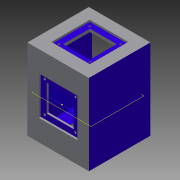
# Autodesk Inventor part: brain box bottom
Saved by Autodesk Inventor 2015 (Build 190159000, 159)
## iProperties
Created: 2014-09-09
Part Number: brain box bottom
Material: Generic
Document SubType Name: Modeling
Designer: ericd_000
Density: 1 g/cm^3
Appearance: Default
Author: ericd_000
Autodesk Inventor part; units mm, degrees
ref_plane "YZ Plane" through (0, 0, 0) normal (1, 0, 0) x (0, 1, 0)
ref_plane "XZ Plane" through (0, 0, 0) normal (0, 1, 0) x (-1, 0, 0)
ref_plane "XY Plane" through (0, 0, 0) normal (0, 0, 1) x (1, 0, 0)
sketch "Sketch1" plane through (0, 0, 0) normal (0, 1, 0) x (-1, 0, 0)
  line L0 (80, 100) -> (-80, 100)
  line L1 (-80, 100) -> (-80, -100)
  line L2 (-80, -100) -> (80, -100)
  line L3 (80, -100) -> (80, 100)
  point P0 (0, 0)
  point P1 (80, 0)
  point P2 (0, -100)
  dimension "d0" = 200
  dimension "d1" = 160
  constraints: 8 end point, 2 midpoint, 2 parallel, 1 horizontal, 1 horizontal alignment, 1 perpendicular, 1 vertical alignment
  measures "d0" distance of L2.end L0.start
  measures "d1" distance of L0.start L0.end
extrude "Extrusion1" add sketch "Sketch1" along normal blind 5
sketch "Sketch2" plane through (0, 5, 0) normal (0, 1, 0) x (1, 0, 0)
  line L0 (-80, -100) -> (80, -100)
  line L1 (80, -100) -> (80, 100)
  line L2 (80, 100) -> (-80, 100)
  line L3 (-80, 100) -> (-80, -100)
  line L4 (-72, -92) -> (72, -92)
  line L5 (72, -92) -> (72, 92)
  line L6 (72, 92) -> (-72, 92)
  line L7 (-72, 92) -> (-72, -92)
  point P0 (0, 0)
  dimension "d4" = 8
  constraints: 16 end point, 4 parallel, 2 perpendicular, 1 horizontal, 3 other
  measures "d4" distance between parallel lines of L3 L7
extrude "Extrusion2" add sketch "Sketch2" along normal blind 150
sketch "Sketch3" plane through (0, 155, 0) normal (0, 1, 0) x (1, 0, 0)
  circle A0 centre (-76, 96) radius 1.5
  circle A1 centre (76, 96) radius 1.5
  circle A2 centre (76, -96) radius 1.5
  circle A3 centre (-76, -96) radius 1.5
  line L0 (80, -100) -> (80, 100) projected
  line L1 (-80, -100) -> (80, -100) projected
  line L2 (80, 100) -> (-80, 100) projected
  line L3 (-80, 100) -> (-80, -100) projected
  point P0 (0, 0)
  dimension "d8" = 3
  dimension "d12" = 4
  dimension "d16" = 4
  dimension "d18" = 3
  dimension "d19" = 4
  dimension "d20" = 4
  dimension "d21" = 3
  dimension "d22" = 4
  dimension "d23" = 4
  dimension "d24" = 4
  dimension "d25" = 4
  dimension "d26" = 3
  constraints: 4 centre point
  measures "d8" diameter of A1
  measures "d12" distance from line of A1.centre L0
  measures "d16" distance from line of L2 A1.centre
  measures "d18" diameter of A0
  measures "d19" distance from line of L3 A0.centre
  measures "d20" distance from line of L2 A0.centre
  measures "d21" diameter of A2
  measures "d22" distance from line of L0 A2.centre
  measures "d23" distance from line of L1 A2.centre
  measures "d24" distance from line of L3 A3.centre
  measures "d25" distance from line of A3.centre L1
  measures "d26" diameter of A3
extrude "Extrusion3" cut sketch "Sketch3" against normal blind 15 contours A0 | A1 | A2 | A3
sketch "Sketch4" plane through (80, 0, 100) normal (1, 0, 0) x (0, 0, -1)
  line L0 (50, 127.5) -> (150, 127.5)
  line L1 (150, 127.5) -> (150, 27.5)
  line L2 (150, 27.5) -> (50, 27.5)
  line L3 (50, 27.5) -> (50, 127.5)
  line L4 (0, 155) -> (200, 155) projected
  line L5 (200, 0) -> (200, 155) projected
  point P0 (100, 0)
  point P1 (100, 127.5)
  point P2 (100, 155)
  point P3 (150, 77.5)
  point P4 (200, 77.5)
  dimension "d29" = 100
  dimension "d30" = 100
  constraints: 8 end point, 4 midpoint, 2 parallel, 1 horizontal, 1 horizontal alignment, 1 perpendicular, 1 vertical alignment
  measures "d29" distance of L0.start L0.end
  measures "d30" distance of L2.end L0.start
sketch "Sketch5" plane through (-80, 0, 100) normal (0, 0, 1) x (1, 0, 0)
  line L0 (45, 112.5) -> (115, 112.5)
  line L1 (115, 112.5) -> (115, 42.5)
  line L2 (115, 42.5) -> (45, 42.5)
  line L3 (45, 42.5) -> (45, 112.5)
  line L4 (160, 0) -> (160, 155) projected
  line L5 (0, 155) -> (160, 155) projected
  point P0 (80, 0)
  point P1 (115, 77.5)
  point P2 (160, 77.5)
  point P3 (80, 112.5)
  point P4 (80, 155)
  dimension "d31" = 70
  dimension "d32" = 70
  constraints: 8 end point, 4 midpoint, 2 parallel, 1 horizontal, 1 horizontal alignment, 1 perpendicular, 1 vertical alignment
  measures "d31" distance of L0.start L0.end
  measures "d32" distance of L0.end L1.end
extrude "Extrusion4" cut sketch "Sketch5" against normal blind 10
sketch "Sketch6" plane through (-80, 0, 100) normal (0, 0, 1) x (1, 0, 0)
  line L0 (45, 112.5) -> (115, 112.5)
  line L1 (115, 112.5) -> (115, 42.5)
  line L2 (115, 42.5) -> (45, 42.5)
  line L3 (45, 42.5) -> (45, 112.5)
  line L4 (30, 127.5) -> (130, 127.5)
  line L5 (130, 127.5) -> (130, 27.5)
  line L6 (130, 27.5) -> (30, 27.5)
  line L7 (30, 27.5) -> (30, 127.5)
  circle A0 centre (40, 117.5) radius 2.75
  circle A1 centre (40, 37.5) radius 2.75
  circle A2 centre (120, 117.5) radius 2.75
  circle A3 centre (120, 37.5) radius 2.75
  point P0 (80, 0)
  dimension "d35" = 15
  dimension "d36" = 10
  dimension "d37" = 10
  dimension "d38" = 5.5
  dimension "d41" = 80
  dimension "d44" = 80
  constraints: 16 end point, 4 centre point, 4 parallel, 2 horizontal, 2 perpendicular, 1 vertical, 9 other
  measures "d35" distance between parallel lines of L4 L0
  measures "d36" distance from line of L7 A0.centre
  measures "d37" distance from line of L4 A0.centre
  measures "d38" diameter of A0
  measures "d41" distance of A0.centre A1.centre
  measures "d44" distance of A0.centre A2.centre
extrude "Extrusion5" cut sketch "Sketch6" against normal blind 8 contours A0 | A1 | A2 | A3
sketch "Sketch7" plane through (0, 5, 0) normal (0, 1, 0) x (1, 0, 0)
  line L0 (72, 92) -> (72, -92) construction
  line L1 (72, 0) -> (-72, 0) construction
  line L2 (-72, -92) -> (-72, 92) construction
  point P0 (0, 0)
  constraints: 2 end point, 2 midpoint
ref_plane "Work Plane1" through (72, 5, 0) normal (0, 0, -1) x (-1, 0, 0)
mirror "Mirror1" about plane through (72, 5, 0) normal (0, 0, -1) of "Extrusion5"
mirror "Mirror2" about plane through (72, 5, 0) normal (0, 0, -1) of "Extrusion4"
sketch "Sketch8" plane through (0, 0, 0) normal (0, -1, 0) x (1, 0, 0)
  line L0 (35, -35) -> (-35, -35)
  line L1 (-35, -35) -> (-35, 35)
  line L2 (-35, 35) -> (35, 35)
  line L3 (35, 35) -> (35, -35)
  line L4 (50, -50) -> (-50, -50)
  line L5 (-50, -50) -> (-50, 50)
  line L6 (-50, 50) -> (50, 50)
  line L7 (50, 50) -> (50, -50)
  circle A0 centre (40, -40) radius 2.75
  circle A1 centre (40, 40) radius 2.75
  circle A2 centre (-40, -40) radius 2.75
  circle A3 centre (-40, 40) radius 2.75
  point P0 (0, 0)
  point P1 (-35, 0)
  point P2 (0, -35)
  dimension "d50" = 70
  dimension "d51" = 70
  dimension "d52" = 15
  dimension "d53" = 5.5
  dimension "d54" = 10
  dimension "d55" = 10
  dimension "d58" = 80
  dimension "d65" = 80
  constraints: 16 end point, 4 centre point, 4 parallel, 2 horizontal, 2 midpoint, 2 perpendicular, 1 horizontal alignment, 1 vertical, 1 vertical alignment, 9 other
  measures "d50" distance of L0.start L0.end
  measures "d51" distance of L0.end L1.end
  measures "d52" distance between parallel lines of L7 L3
  measures "d53" diameter of A0
  measures "d54" distance from line of L7 A0.centre
  measures "d55" distance from line of L4 A0.centre
  measures "d58" distance of A0.centre A1.centre
  measures "d65" distance of A0.centre A2.centre
extrude "Extrusion6" cut sketch "Sketch8" against normal blind 8 contours L0 L1 L2 L3 | A0 | A1 | A2 | A3
sketch "Sketch10" plane through (80, 0, -100) normal (0, 0, -1) x (-1, 0, 0)
  line L0 (130, 127.5) -> (30, 127.5)
  line L1 (30, 127.5) -> (30, 27.5)
  line L2 (30, 27.5) -> (130, 27.5)
  line L3 (130, 27.5) -> (130, 127.5)
  line L4 (0, 155) -> (160, 155) projected
  line L5 (115, 112.5) -> (115, 42.5) projected
  line L6 (115, 42.5) -> (45, 42.5) projected
  line L7 (160, 155) -> (0, 155)
  line L8 (0, 155) -> (0, 0)
  line L9 (0, 0) -> (160, 0)
  line L10 (160, 0) -> (160, 155)
  point P0 (80, 0)
  point P1 (130, 77.5)
  point P2 (115, 77.5)
  point P3 (80, 27.5)
  point P4 (80, 42.5)
  dimension "d72" = 100
  dimension "d73" = 100
  constraints: 16 end point, 4 midpoint, 4 parallel, 2 horizontal, 2 perpendicular, 1 horizontal alignment, 1 vertical alignment
  measures "d72" distance of L2.end L0.start
  measures "d73" distance of L1.end L2.end
extrude "Extrusion7" add sketch "Sketch10" along normal blind 5
mirror "Mirror3" about plane through (72, 5, 0) normal (0, 0, -1) of "Extrusion7"
sketch "Sketch11" plane through (0, 0, 0) normal (0, -1, 0) x (1, 0, 0)
  line L0 (50, 50) -> (-50, 50)
  line L1 (-50, 50) -> (-50, -50)
  line L2 (-50, -50) -> (50, -50)
  line L3 (50, -50) -> (50, 50)
  line L4 (35, 35) -> (35, -35) projected
  line L5 (35, -35) -> (-35, -35) projected
  line L6 (80, 105) -> (-80, 105)
  line L7 (-80, 105) -> (-80, -105)
  line L8 (-80, -105) -> (80, -105)
  line L9 (80, -105) -> (80, 105)
  point P0 (0, 0)
  point P1 (50, 0)
  point P2 (35, 0)
  point P3 (0, -50)
  point P4 (0, -35)
  dimension "d77" = 100
  dimension "d78" = 100
  constraints: 16 end point, 4 midpoint, 4 parallel, 2 horizontal, 2 perpendicular, 1 horizontal alignment, 1 vertical alignment
  measures "d77" distance of L2.end L0.start
  measures "d78" distance of L1.end L2.end
extrude "Extrusion8" add sketch "Sketch11" along normal blind 5
body "Solid1"
